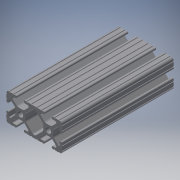
# Autodesk Inventor part: 4in_1020
Saved by Autodesk Inventor 2019 (Build 230136000, 136)
## iProperties
Company: 80/20 Inc.
Created: 2014-04-23
Part Number: 4in_1020
Material: Generic
Document SubType Name: Modeling
Density: 1 g/cm^3
Vendor: 80/20 Inc.
Engineer: Ross Bowman
Designer: Ross Bowman
Catalog Web Link: 8020.net
Appearance: Default
Material: 6105-T5 Aluminum
Author: Ross Bowman
Keywords: 80/20 , 8020 , T-Slot , Extrusion
Autodesk Inventor part; units mm, degrees
ref_plane "YZ Plane" through (0, 0, 0) normal (1, 0, 0) x (0, 1, 0)
ref_plane "XZ Plane" through (0, 0, 0) normal (0, 1, 0) x (-1, 0, 0)
ref_plane "XY Plane" through (0, 0, 0) normal (0, 0, 1) x (1, 0, 0)
sketch "Sketch1" plane through (0, 0, 0) normal (0, 0, 1) x (1, 0, 0)
  line L0 (7.2595, 3.8694) -> (1.5457, 9.5728)
  arc A0 (1.5457, 9.5728) -> (0.4332, 10.033) centre (0.4332, 8.4582) ccw
  line L1 (0.4332, 10.033) -> (-0.4332, 10.033)
  arc A1 (-0.4332, 10.033) -> (-1.5457, 9.5728) centre (-0.4332, 8.4582) ccw
  line L2 (-1.5457, 9.5728) -> (-7.2595, 3.8694)
  arc A2 (-7.2595, 3.8694) -> (-8.1915, 1.6223) centre (-5.0165, 1.6223) ccw
  line L3 (-8.1915, 1.6223) -> (-8.1915, -1.6223)
  line L4 (-7.2829, -3.8459) -> (-1.6756, -9.5611)
  arc A3 (-1.6756, -9.5611) -> (-0.5515, -10.033) centre (-0.5515, -8.4582) ccw
  line L5 (-0.5515, -10.033) -> (0.3952, -10.033)
  arc A4 (0.3952, -10.033) -> (1.504, -9.5765) centre (0.3952, -8.4582) ccw
  line L6 (1.504, -9.5765) -> (7.252, -3.8768)
  arc A5 (7.252, -3.8768) -> (8.1915, -1.6223) centre (5.0165, -1.6223) ccw
  line L7 (8.1915, -1.6223) -> (8.1915, 1.6223)
  arc A6 (8.1915, 1.6223) -> (7.2595, 3.8694) centre (5.0165, 1.6223) ccw
  circle A7 centre (12.7, 0) radius 2.6035
  circle A8 centre (-12.7, 0) radius 2.6035
  arc A9 (-8.1915, -1.6223) -> (-7.2829, -3.8459) centre (-5.0165, -1.6223) ccw
  line L8 (-15.9385, -11.651) -> (-15.9385, -11.5392)
  arc A10 (-15.9385, -11.5392) -> (-16.9875, -10.4902) centre (-16.9875, -11.5392) ccw
  line L9 (-16.9875, -10.4902) -> (-19.1164, -10.4902)
  arc A11 (-19.8441, -8.7652) -> (-19.1164, -10.4902) centre (-19.1164, -9.4742) ccw
  line L10 (-19.8441, -8.7652) -> (-16.619, -5.4551)
  arc A12 (-14.3449, -4.4958) -> (-16.619, -5.4551) centre (-14.3449, -7.6708) ccw
  line L11 (-14.3449, -4.4958) -> (-11.0833, -4.4958)
  arc A13 (-8.817, -5.4472) -> (-11.0833, -4.4958) centre (-11.0833, -7.6708) ccw
  line L12 (-8.817, -5.4472) -> (-5.5642, -8.7627)
  arc A14 (-6.2894, -10.4902) -> (-5.5642, -8.7627) centre (-6.2894, -9.4742) ccw
  line L13 (-6.2894, -10.4902) -> (-8.4125, -10.4902)
  arc A15 (-8.4125, -10.4902) -> (-9.4615, -11.5392) centre (-8.4125, -11.5392) ccw
  line L14 (-9.4615, -11.5392) -> (-9.4615, -11.6511)
  arc A16 (-9.4615, -11.6511) -> (-8.4125, -12.7) centre (-8.4125, -11.651) ccw
  line L15 (-8.4125, -12.7) -> (-7.3829, -12.7)
  arc A17 (-6.3669, -12.7) -> (-7.3829, -12.7) centre (-6.8749, -12.7) ccw
  line L16 (-6.3669, -12.7) -> (-3.1496, -12.7)
  arc A18 (-2.1336, -12.7) -> (-3.1496, -12.7) centre (-2.6416, -12.7) ccw
  line L17 (-2.1336, -12.7) -> (2.1336, -12.7)
  arc A19 (3.1496, -12.7) -> (2.1336, -12.7) centre (2.6416, -12.7) ccw
  line L18 (3.1496, -12.7) -> (6.3669, -12.7)
  arc A20 (7.3829, -12.7) -> (6.3669, -12.7) centre (6.8749, -12.7) ccw
  line L19 (7.3829, -12.7) -> (8.4126, -12.7)
  arc A21 (8.4126, -12.7) -> (9.4615, -11.651) centre (8.4125, -11.651) ccw
  line L20 (9.4615, -11.651) -> (9.4615, -11.5392)
  arc A22 (9.4615, -11.5392) -> (8.4125, -10.4902) centre (8.4125, -11.5392) ccw
  line L21 (8.4125, -10.4902) -> (6.2836, -10.4902)
  arc A23 (5.5326, -8.6661) -> (6.2836, -10.4902) centre (6.2836, -9.4235) ccw
  line L22 (5.5326, -8.6661) -> (8.81, -5.4163)
  arc A24 (11.0455, -4.4958) -> (8.81, -5.4163) centre (11.0455, -7.6708) ccw
  line L23 (11.0455, -4.4958) -> (14.3545, -4.4958)
  arc A25 (16.59, -5.4163) -> (14.3545, -4.4958) centre (14.3545, -7.6708) ccw
  line L24 (16.59, -5.4163) -> (19.8674, -8.6661)
  arc A26 (19.1164, -10.4902) -> (19.8674, -8.6661) centre (19.1164, -9.4235) ccw
  line L25 (19.1164, -10.4902) -> (16.9875, -10.4902)
  arc A27 (16.9875, -10.4902) -> (15.9385, -11.5392) centre (16.9875, -11.5392) ccw
  line L26 (15.9385, -11.5392) -> (15.9385, -11.651)
  arc A28 (15.9385, -11.651) -> (16.9874, -12.7) centre (16.9875, -11.651) ccw
  line L27 (16.9874, -12.7) -> (18.0171, -12.7)
  arc A29 (19.0331, -12.7) -> (18.0171, -12.7) centre (18.5251, -12.7) ccw
  line L28 (19.0331, -12.7) -> (22.2504, -12.7)
  arc A30 (23.2664, -12.6998) -> (22.2504, -12.7) centre (22.7584, -12.7) ccw
  arc A31 (23.2664, -12.6998) -> (25.3998, -10.5664) centre (23.2918, -10.5918) ccw
  arc A32 (25.4, -9.5504) -> (25.3998, -10.5664) centre (25.4, -10.0584) ccw
  line L29 (25.4, -9.5504) -> (25.4, -6.3331)
  arc A33 (25.4, -5.3171) -> (25.4, -6.3331) centre (25.4, -5.8251) ccw
  line L30 (25.4, -5.3171) -> (25.4, -4.2375)
  arc A34 (25.4, -4.2375) -> (24.401, -3.2385) centre (24.401, -4.2375) ccw
  line L31 (24.401, -3.2385) -> (24.2392, -3.2385)
  arc A35 (24.2392, -3.2385) -> (23.1902, -4.2875) centre (24.2392, -4.2875) ccw
  line L32 (23.1902, -4.2875) -> (23.1902, -6.3347)
  arc A36 (21.434, -7.0665) -> (23.1902, -6.3347) centre (22.1596, -6.3347) ccw
  line L33 (21.434, -7.0665) -> (18.148, -3.8082)
  arc A37 (17.2085, -1.5536) -> (18.148, -3.8082) centre (20.3835, -1.5536) ccw
  line L34 (17.2085, -1.5536) -> (17.2085, 1.6952)
  arc A38 (18.1405, 3.9423) -> (17.2085, 1.6952) centre (20.3835, 1.6952) ccw
  line L35 (18.1405, 3.9423) -> (21.4316, 7.2274)
  arc A39 (23.1902, 6.498) -> (21.4316, 7.2274) centre (22.1596, 6.498) ccw
  line L36 (23.1902, 6.498) -> (23.1902, 4.2875)
  arc A40 (23.1902, 4.2875) -> (24.2392, 3.2385) centre (24.2392, 4.2875) ccw
  line L37 (24.2392, 3.2385) -> (24.351, 3.2385)
  arc A41 (24.351, 3.2385) -> (25.4, 4.2875) centre (24.351, 4.2875) ccw
  line L38 (25.4, 4.2875) -> (25.4, 5.3171)
  arc A42 (25.4, 6.3331) -> (25.4, 5.3171) centre (25.4, 5.8251) ccw
  line L39 (25.4, 6.3331) -> (25.4, 9.5504)
  arc A43 (25.3998, 10.5664) -> (25.4, 9.5504) centre (25.4, 10.0584) ccw
  arc A44 (25.3998, 10.5664) -> (23.2664, 12.6998) centre (23.2918, 10.5918) ccw
  arc A45 (22.2504, 12.7) -> (23.2664, 12.6998) centre (22.7584, 12.7) ccw
  line L40 (22.2504, 12.7) -> (19.0331, 12.7)
  arc A46 (18.0171, 12.7) -> (19.0331, 12.7) centre (18.5251, 12.7) ccw
  line L41 (18.0171, 12.7) -> (16.9875, 12.7)
  arc A47 (16.9875, 12.7) -> (15.9384, 11.651) centre (16.9875, 11.651) ccw
  line L42 (15.9384, 11.651) -> (15.9384, 11.5392)
  arc A48 (15.9384, 11.5392) -> (16.9875, 10.4902) centre (16.9875, 11.5392) ccw
  line L43 (16.9875, 10.4902) -> (19.1164, 10.4902)
  arc A49 (19.8341, 8.7551) -> (19.1164, 10.4902) centre (19.1164, 9.4742) ccw
  line L44 (19.8341, 8.7551) -> (16.4966, 5.4237)
  arc A50 (14.2536, 4.4958) -> (16.4966, 5.4237) centre (14.2536, 7.6708) ccw
  line L45 (14.2536, 4.4958) -> (11.1464, 4.4958)
  arc A51 (8.9034, 5.4237) -> (11.1464, 4.4958) centre (11.1464, 7.6708) ccw
  line L46 (8.9034, 5.4237) -> (5.5659, 8.7551)
  arc A52 (6.2836, 10.4902) -> (5.5659, 8.7551) centre (6.2836, 9.4742) ccw
  line L47 (6.2836, 10.4902) -> (8.4125, 10.4902)
  arc A53 (8.4125, 10.4902) -> (9.4615, 11.5392) centre (8.4125, 11.5392) ccw
  line L48 (9.4615, 11.5392) -> (9.4615, 11.651)
  arc A54 (9.4615, 11.651) -> (8.4125, 12.7) centre (8.4125, 11.651) ccw
  line L49 (8.4125, 12.7) -> (7.3829, 12.7)
  arc A55 (6.3669, 12.7) -> (7.3829, 12.7) centre (6.8749, 12.7) ccw
  line L50 (6.3669, 12.7) -> (3.1496, 12.7)
  arc A56 (2.1336, 12.7) -> (3.1496, 12.7) centre (2.6416, 12.7) ccw
  line L51 (2.1336, 12.7) -> (-2.1336, 12.7)
  arc A57 (-3.1496, 12.7) -> (-2.1336, 12.7) centre (-2.6416, 12.7) ccw
  line L52 (-3.1496, 12.7) -> (-6.3669, 12.7)
  arc A58 (-7.3829, 12.7) -> (-6.3669, 12.7) centre (-6.8749, 12.7) ccw
  line L53 (-7.3829, 12.7) -> (-8.4125, 12.7)
  arc A59 (-8.4125, 12.7) -> (-9.4616, 11.651) centre (-8.4125, 11.651) ccw
  line L54 (-9.4616, 11.651) -> (-9.4616, 11.5392)
  arc A60 (-9.4616, 11.5392) -> (-8.4125, 10.4902) centre (-8.4125, 11.5392) ccw
  line L55 (-8.4125, 10.4902) -> (-6.2894, 10.4902)
  arc A61 (-5.4807, 8.5353) -> (-6.2894, 10.4902) centre (-6.2894, 9.3455) ccw
  line L56 (-5.4807, 8.5353) -> (-8.5979, 5.4237)
  arc A62 (-10.8409, 4.4958) -> (-8.5979, 5.4237) centre (-10.8409, 7.6708) ccw
  line L57 (-10.8409, 4.4958) -> (-14.1026, 4.4958)
  arc A63 (-16.1879, 5.2766) -> (-14.1026, 4.4958) centre (-14.1026, 7.6708) ccw
  line L58 (-16.1879, 5.2766) -> (-19.8682, 8.4822)
  arc A64 (-19.1164, 10.4902) -> (-19.8682, 8.4822) centre (-19.1164, 9.3455) ccw
  line L59 (-19.1164, 10.4902) -> (-16.9875, 10.4902)
  arc A65 (-16.9875, 10.4902) -> (-15.9384, 11.5392) centre (-16.9875, 11.5392) ccw
  line L60 (-15.9384, 11.5392) -> (-15.9384, 11.651)
  arc A66 (-15.9384, 11.651) -> (-16.9875, 12.7) centre (-16.9875, 11.651) ccw
  line L61 (-16.9875, 12.7) -> (-18.0171, 12.7)
  arc A67 (-19.0331, 12.7) -> (-18.0171, 12.7) centre (-18.5251, 12.7) ccw
  line L62 (-19.0331, 12.7) -> (-22.2504, 12.7)
  arc A68 (-23.2664, 12.6998) -> (-22.2504, 12.7) centre (-22.7584, 12.7) ccw
  arc A69 (-23.2664, 12.6998) -> (-25.3998, 10.5664) centre (-23.2918, 10.5918) ccw
  arc A70 (-25.4, 9.5504) -> (-25.3998, 10.5664) centre (-25.4, 10.0584) ccw
  line L63 (-25.4, 9.5504) -> (-25.4, 6.3331)
  arc A71 (-25.4, 5.3171) -> (-25.4, 6.3331) centre (-25.4, 5.8251) ccw
  line L64 (-25.4, 5.3171) -> (-25.4, 4.2375)
  arc A72 (-25.4, 4.2375) -> (-24.401, 3.2385) centre (-24.401, 4.2375) ccw
  line L65 (-24.401, 3.2385) -> (-24.1892, 3.2385)
  arc A73 (-24.1892, 3.2385) -> (-23.1902, 4.2375) centre (-24.1892, 4.2375) ccw
  line L66 (-23.1902, 4.2375) -> (-23.1902, 6.1559)
  arc A74 (-21.584, 6.8869) -> (-23.1902, 6.1559) centre (-22.2207, 6.1559) ccw
  line L67 (-21.584, 6.8869) -> (-18.2982, 4.025)
  arc A75 (-17.2085, 1.6308) -> (-18.2982, 4.025) centre (-20.3835, 1.6308) ccw
  line L68 (-17.2085, 1.6308) -> (-17.2085, -1.6308)
  arc A76 (-18.1094, -3.8465) -> (-17.2085, -1.6308) centre (-20.3835, -1.6308) ccw
  line L69 (-18.1094, -3.8465) -> (-21.5263, -7.3534)
  arc A77 (-23.1902, -6.6769) -> (-21.5263, -7.3534) centre (-22.2207, -6.6769) ccw
  line L70 (-23.1902, -6.6769) -> (-23.1902, -4.2375)
  arc A78 (-23.1902, -4.2375) -> (-24.1892, -3.2385) centre (-24.1892, -4.2375) ccw
  line L71 (-24.1892, -3.2385) -> (-24.401, -3.2385)
  arc A79 (-24.401, -3.2385) -> (-25.4, -4.2375) centre (-24.401, -4.2375) ccw
  line L72 (-25.4, -4.2375) -> (-25.4, -5.3171)
  arc A80 (-25.4, -6.3332) -> (-25.4, -5.3171) centre (-25.4, -5.8251) ccw
  line L73 (-25.4, -6.3332) -> (-25.4, -9.5504)
  arc A81 (-25.3998, -10.5664) -> (-25.4, -9.5504) centre (-25.4, -10.0584) ccw
  arc A82 (-25.3998, -10.5664) -> (-23.2664, -12.6998) centre (-23.2918, -10.5918) ccw
  arc A83 (-22.2504, -12.7) -> (-23.2664, -12.6998) centre (-22.7584, -12.7) ccw
  line L74 (-22.2504, -12.7) -> (-19.0331, -12.7)
  arc A84 (-18.0171, -12.7) -> (-19.0331, -12.7) centre (-18.5251, -12.7) ccw
  line L75 (-18.0171, -12.7) -> (-16.9874, -12.7)
  arc A85 (-16.9874, -12.7) -> (-15.9385, -11.651) centre (-16.9874, -11.651) ccw
  point P0 (0, 0)
  constraints: 168 point on circle, 152 end point, 86 centre point
extrude "Extrusion1" add sketch "Sketch1" against normal blind 101.6
body "Solid1"
